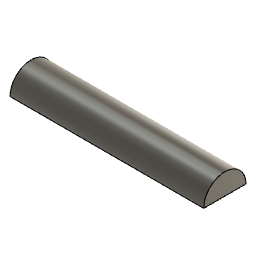
final project 2 v1 (Autodesk Fusion 360 design; units mm, degrees)
Autodesk Fusion 360 part; units mm, degrees
sketch "草图1" plane through (0, 0, 0) normal (0, 0, 1) x (1, 0, 0)
  line L0 (-54.8343, 11.7117) -> (55.1657, 11.7117)
  line L1 (55.1657, 11.7117) -> (55.1657, -0.2883)
  line L2 (55.1657, -0.2883) -> (-54.8343, -0.2883)
  line L3 (-54.8343, -0.2883) -> (-54.8343, 11.7117)
  dimension "d1" = 110
  dimension "d2" = 12
  constraint horizontal L0
  constraint vertical L1
  constraint horizontal L2
  constraint vertical L3
  measures "d1" distance of L0.start L0.end
  measures "d2" distance of L0.start L2.end
revolve "旋转1" add sketch "草图1" angle 180 about axis through (55.1657, -0.2883, 0) along (1, 0, 0)
